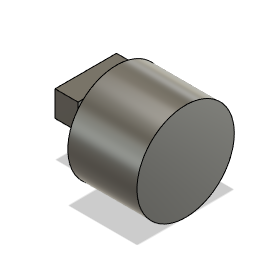
BottomTest v8 (Autodesk Fusion 360 archive; units mm, degrees)
design "StepperAndWheel"
Autodesk Fusion 360 part; units mm, degrees
sketch "草图1" plane through (0, 0, 0) normal (0, 1, 0) x (1, 0, 0)
  line L0 (0, -6) -> (9, -6)
  line L1 (9, -6) -> (9, 18)
  line L2 (9, 18) -> (0, 18)
  line L3 (0, 18) -> (0, -6)
  constraint horizontal L0
  constraint vertical L1
  constraint horizontal L2
  constraint vertical L3
extrude "拉伸1" add sketch "草图1" along normal blind 5 and the other way blind 0
extrude "拉伸2" add 1 faces at (3, 5, -10) along direction (0, 1, 0) blind 5
cylinder "圆柱体基本要素1" add diameter 3 height 9 placed x (0, 0, -1) y (0, 1, 0) z (1, 0, 0) at (9, 5, 0)
cylinder "圆柱体基本要素2" add diameter 38 height 27 placed x (0, 0, -1) y (0, 1, 0) z (1, 0, 0) at (18, 5, 0)

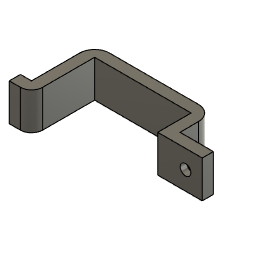
design "StepperMount"
Autodesk Fusion 360 part; units mm, degrees
sketch "草图1" plane through (0, 0, 0) normal (0, 1, 0) x (1, 0, 0)
  line L0 (12, 9) -> (38, 9)
  line L1 (38, 9) -> (38, 0)
  line L2 (38, 0) -> (50, 0)
  line L3 (50, 0) -> (50, 3)
  line L4 (50, 3) -> (41, 3)
  line L5 (41, 3) -> (41, 8)
  line L6 (37, 12) -> (13, 12)
  line L7 (9, -8) -> (6, -8)
  line L8 (6, -8) -> (6, -5)
  line L9 (6, -5) -> (9, -5)
  line L10 (9, 8) -> (9, -5)
  line L11 (12, 9) -> (12, -5)
  arc A0 (9, -8) -> (12, -5) centre (9, -5) ccw
  arc A1 (13, 12) -> (9, 8) centre (13, 8) ccw
  arc A2 (41, 8) -> (37, 12) centre (37, 8) ccw
  dimension "d21" = 3
  dimension "d22" = 4
  constraint perpendicular L0 L1
  constraint perpendicular L1 L2
  constraint perpendicular L2 L3
  constraint perpendicular L3 L4
  constraint perpendicular L4 L5
  constraint perpendicular L5 L6
  constraint perpendicular L7 L8
  constraint perpendicular L8 L9
  constraint perpendicular L9 L10
  constraint perpendicular L0 L11
  constraint tangent L7 A0
  constraint tangent L11 A0
  constraint tangent L6 A1
  constraint tangent L10 A1
  constraint tangent L5 A2
  constraint tangent L6 A2
  constraint equal A1 A2
  measures "d21" radius of A0
  measures "d22" radius of A1
extrude "拉伸1" add sketch "草图1" along normal blind 10
sketch "草图2" plane through (0, 0, -3) normal (0, 0, -1) x (-1, 0, 0)
  line L0 (-9, 0) -> (0, 0)
  line L1 (0, 0) -> (0, 10)
  line L2 (0, 10) -> (-9, 10)
  line L3 (-9, 10) -> (-9, 0)
  circle A0 centre (-4.5, 5) radius 1.5
  dimension "d3" = 3
  measures "d3" diameter of A0
hole "孔1" at (4.5, 5, -3) direction (0, 0, 1) diameter 3 depth 9 tip angle 180
hole "孔2" at (45.5, 5, -3) direction (0, 0, 1) diameter 2.9 depth 10 tip angle 180 countersink diameter 5.3 countersink angle 90
delete_face "删除面1" [no effect]
move_body "移动1" bodies 1 to x (1, 0, 0) y (0, 1, 0) z (0, 0, 1) at (-25, 0, 0)
hole "孔3" at (-20.5, 5, -3) direction (0, 0, 1) diameter 2.9 depth 10 tip angle 180 countersink diameter 5.3 countersink angle 90
